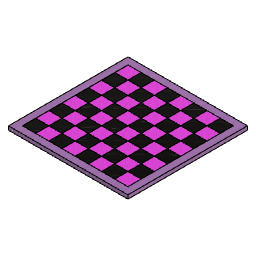
Chess Board black&pink (Autodesk Fusion 360 design; units mm, degrees)
Autodesk Fusion 360 part; units mm, degrees
sketch "Sketch1" plane through (0, 0, 0) normal (0, 0, 1) x (1, 0, 0)
  line L0 (-7, 7) -> (7, 7)
  line L1 (7, 7) -> (7, -7)
  line L2 (7, -7) -> (-7, -7)
  line L3 (-7, -7) -> (-7, 7)
  line L4 (-7, 7) -> (-21, 7)
  line L5 (-21, 7) -> (-21, 21)
  line L6 (-21, 21) -> (-7, 21)
  line L7 (-7, 21) -> (-7, 7)
  dimension "d1" = 14
  dimension "d2" = 14
  constraint horizontal L0
  constraint vertical L1
  constraint horizontal L2
  constraint vertical L3
  constraint horizontal L4
  constraint vertical L5
  constraint horizontal L6
  constraint vertical L7
  measures "d1" distance of L0.start L2.end
  measures "d2" distance of L1.end L2.end
extrude "Extrude1" add sketch "Sketch1" along normal blind 4 makes body 1
pattern_linear "R-Pattern1" count 4 spacing 28 along (0, -1, 0) count 4 spacing 28 along (1, 0, 0) of bodies 1 makes body 2 at (-11.6667, -16.3333, 0) makes body 3 at (-11.6667, -44.3333, 0) makes body 4 at (-11.6667, -72.3333, 0) makes body 5 at (16.3333, 11.6667, 0) makes body 6 at (16.3333, -16.3333, 0) makes body 7 at (16.3333, -44.3333, 0) makes body 8 at (16.3333, -72.3333, 0) makes body 9 at (44.3333, 11.6667, 0) makes body 10 at (44.3333, -16.3333, 0) makes body 11 at (44.3333, -44.3333, 0) makes body 12 at (44.3333, -72.3333, 0) makes body 13 at (72.3333, 11.6667, 0) makes body 14 at (72.3333, -16.3333, 0) makes body 15 at (72.3333, -44.3333, 0) makes body 16 at (72.3333, -72.3333, 0)
combine "Combine1" operation add target body 14 tool bodies 8 9 13 12 10 11 4 16 3 6 7 15 5 2 1
copy_body "CopyPasteBodies1" bodies 14 makes body 17
move_body "Move1" bodies 17 to x (0, -1, 0) y (1, 0, 0) z (0, 0, 1) at (70, 0, 0)
sketch "Sketch2" plane through (0, 0, 0) normal (0, 0, 1) x (1, 0, 0)
  line L0 (-20.858, -91) -> (91, -91)
  line L1 (91, -91) -> (91, 21)
  line L2 (91, 21) -> (-20.858, 21)
  line L3 (-20.858, 21) -> (-20.858, -91)
  line L4 (-7, -91) -> (-21, -91)
  line L5 (-28.3436, 28.4857) -> (-28.3436, -98.4857)
  line L6 (-28.3436, -98.4857) -> (98.4857, -98.4857)
  line L7 (98.4857, -98.4857) -> (98.4857, 28.4857)
  line L8 (98.4857, 28.4857) -> (-28.3436, 28.4857)
  dimension "d9" = 7.4857
  constraint horizontal L0
  constraint vertical L1
  constraint horizontal L2
  constraint vertical L3
  constraint coincident L0.start L4
extrude "Extrude2" add sketch "Sketch2" along normal blind 4 separate body makes body 18
named bodies: "Chess board pink", "Chess board black", "Chess board purple"
